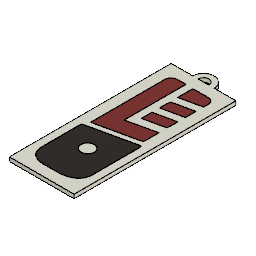
LFE (Autodesk Fusion 360 design; units mm, degrees)
Autodesk Fusion 360 part; units mm, degrees
note: some values were not read from the file. Chosen so that the rebuilt part matches the saved one: which bodies a step acts on. Set by a fixed rule: which sketch regions a step uses.
sketch "Sketch1" plane through (0, 0, 0) normal (0, 0, 1) x (1, 0, 0)
  line L0 (22.7542, -86.2542) -> (47.625, -80.8514)
  line L1 (47.625, -80.8514) -> (52.6521, -79.7322)
  line L2 (52.6521, -79.7322) -> (54.7635, -78.957)
  line L3 (54.7635, -78.957) -> (55.0333, -76.9938)
  line L4 (55.0333, -76.9938) -> (55.0333, -67.4688)
  line L5 (55.0333, -67.4688) -> (50.0063, -68.6382)
  line L6 (50.0063, -68.6382) -> (33.8667, -72.2313)
  line L7 (33.8667, -72.2313) -> (33.8667, -26.1938)
  line L8 (33.8667, -26.1938) -> (28.8396, -26.1938)
  spline S0 degree 3 poles (28.8396, -26.1938) (27.5564, -26.1964) (26.3049, -26.2176) (25.1354, -26.8393) knots 0 0 0 0 1 1 1 1
  spline S1 degree 3 poles (25.1354, -26.8393) (23.2675, -27.8315) (22.7648, -29.5196) (22.7542, -31.4854) knots 0 0 0 0 1 1 1 1
  line L9 (22.7542, -31.4854) -> (22.7542, -40.2167)
  line L10 (22.7542, -40.2167) -> (22.7542, -86.2542)
  line L11 (39.1583, -26.4583) -> (39.1583, -37.8354)
  line L12 (39.1583, -37.8354) -> (55.0333, -34.3958)
  spline S2 degree 3 poles (55.0333, -34.3958) (55.0333, -32.8057) (55.3006, -29.8979) (54.5015, -28.575) knots 0 0 0 0 1 1 1 1
  spline S3 degree 3 poles (54.5015, -28.575) (53.4485, -26.8314) (52.1626, -26.4689) (50.2708, -26.4583) knots 0 0 0 0 1 1 1 1
  line L13 (50.2708, -26.4583) -> (39.1583, -26.4583)
  line L14 (39.1583, -51.3292) -> (55.0333, -47.8896)
  line L15 (55.0333, -47.8896) -> (55.0333, -39.9521)
  line L16 (55.0333, -39.9521) -> (43.9208, -42.3016)
  line L17 (43.9208, -42.3016) -> (39.5737, -43.434)
  line L18 (39.5737, -43.434) -> (39.1583, -45.5083)
  line L19 (39.1583, -45.5083) -> (39.1583, -51.3292)
  line L20 (39.1583, -56.8854) -> (39.1583, -64.8229)
  line L21 (39.1583, -64.8229) -> (50.5354, -62.4099)
  line L22 (50.5354, -62.4099) -> (54.6179, -61.341)
  line L23 (54.6179, -61.341) -> (55.0333, -59.2667)
  line L24 (55.0333, -59.2667) -> (55.0333, -53.4458)
  line L25 (55.0333, -53.4458) -> (50.5354, -54.393)
  line L26 (50.5354, -54.393) -> (39.1583, -56.8854)
  line L27 (56.3404, -82.7114) -> (45.5083, -85.0847)
  line L28 (45.5083, -85.0847) -> (28.575, -88.8074)
  line L29 (28.575, -88.8074) -> (22.7542, -90.1118)
  spline S4 degree 3 poles (22.7542, -90.1118) (22.1377, -90.2467) (21.0344, -90.3711) (20.6428, -90.9002) knots 0 0 0 0 1 1 1 1
  spline S5 degree 3 poles (20.6428, -90.9002) (20.3121, -91.35) (20.3729, -92.3184) (20.3729, -92.8688) knots 0 0 0 0 1 1 1 1
  line L30 (20.3729, -92.8688) -> (20.3729, -112.9771)
  spline S6 degree 3 poles (20.3729, -112.9771) (20.3729, -116.2817) (20.0766, -121.322) (21.1905, -124.3542) knots 0 0 0 0 1 1 1 1
  spline S7 degree 3 poles (21.1905, -124.3542) (22.7991, -128.733) (27.0828, -130.6512) (31.4854, -130.7042) knots 0 0 0 0 1 1 1 1
  spline S8 degree 3 poles (31.4854, -130.7042) (35.8828, -130.7544) (45.1088, -131.1222) (48.9479, -129.9025) knots 0 0 0 0 1 1 1 1
  spline S9 degree 3 poles (48.9479, -129.9025) (53.9194, -128.3229) (57.4066, -125.005) (57.4146, -119.5917) knots 0 0 0 0 1 1 1 1
  line L31 (57.4146, -119.5917) -> (57.4146, -107.6854)
  line L32 (57.4146, -107.6854) -> (57.4146, -88.6354)
  line L33 (57.4146, -88.6354) -> (57.4146, -84.9313)
  spline S10 degree 3 poles (57.4146, -84.9313) (57.4146, -84.4285) (57.4754, -83.3729) (57.1447, -82.9839) knots 0 0 0 0 1 1 1 1
  spline S11 degree 3 poles (57.1447, -82.9839) (56.851, -82.6373) (56.4568, -82.7273) (56.3404, -82.7114) knots 0 0 0 0 1 1 1 1
  spline S12 degree 3 poles (37.5708, -99.3061) (38.6133, -99.2002) (39.5076, -99.2267) (40.4813, -99.6871) knots 0 0 0 0 1 1 1 1
  spline S13 degree 3 poles (40.4813, -99.6871) (45.4766, -102.0498) (43.6033, -109.3682) (38.1, -108.9819) knots 0 0 0 0 1 1 1 1
  spline S14 degree 3 poles (38.1, -108.9819) (32.6469, -108.6009) (31.7341, -100.7401) (37.5708, -99.3061) knots 0 0 0 0 1 1 1 1
  line L34 (14.7542, -18.1937) -> (63.0333, -18.1937)
  line L35 (63.0333, -18.1937) -> (63.0333, -138.7945)
  line L36 (63.0333, -138.7945) -> (14.7542, -138.7945)
  line L37 (14.7542, -138.7945) -> (14.7542, -18.1937)
  line L38 (38.0274, -130.7945) -> (16, -130.7945) construction
  circle A0 centre (38.8938, -18.1937) radius 8
  circle A1 centre (38.8938, -18.1937) radius 4
  dimension "d3" = 8
  dimension "d4" = 8
  dimension "d5" = 8
  dimension "d6" = 8
  dimension "d13" = 16
  dimension "d14" = -4
  constraint horizontal L34
  constraint vertical L35
  constraint horizontal L36
  constraint vertical L37
  constraint coincident S8 L38.start
  constraint horizontal L38
  constraint midpoint L34 A0.centre
  measures "d3" distance of L8 L34
  measures "d4" distance of L15 L35
  measures "d5" distance of L10 L37
  measures "d13" diameter of A0
extrude "Extrude1" add sketch "Sketch1" against normal blind 0.6 contours L0 L1 L2 L3 L4 L5 L6 L7 L8 S0 S1 L9 L10 | L11 L12 S2 S3 L13 | L14 L15 L16 L17 L18 L19 | L20 L21 L22 L23 L24 L25 L26 | L27 L28 L29 S4 S5 L30 S6 S7 S8 S9 L31 L32 L33 S10 S11 makes body 1 at (46.0375, -47.1734, 0) makes body 2 at (48.1542, -32.8965, 0) makes body 3 at (46.7431, -57.8961, 0) makes body 4 at (26.4583, -63.3236, 0) makes body 5 at (52.7338, -102.7556, 0)
extrude "Extrude4" add sketch "Sketch1" against normal blind 3 separate body contours L0 L1 L2 L3 L4 L5 L6 L7 L8 S0 S1 L9 L10 | L11 L12 S2 S3 L13 | L14 L15 L16 L17 L18 L19 | L20 L21 L22 L23 L24 L25 L26 | L27 L28 L29 S4 S5 L30 S6 S7 S8 S9 L31 L32 L33 S10 S11 | S12 S13 S14 | L34 A0 A1 | L34 A1 | L34 A0 A1 | L34 L35 L36 L37 A0 picked at (40.0397, -19.5366) makes body 6
combine "Combine1" operation cut target body 6 tool bodies 5 4 3 2 1 keep tools
ref_plane "WorkPlane1" through (38.776, -106.8798, -0.6) normal (0, 0, 1) x (1, 0, 0)
split "Split1" by plane through (38.776, -106.8798, -0.6) normal (0, 0, 1) bodies 6 makes body 7 at (39.6032, -136.119, 0) makes body 8 at (38.5531, -102.8878, 0)
combine "Combine2" operation add target body 6 tool bodies 7
named bodies: "LFE_keychain_tag_2", "LFE_keychain_tag_1", "LFE_keychain_tag_3", "LFE_keychain_tag_4", "LFE_keychain_tag_5", "LFE_keychain_tag_6", "LFE_keychain_tag_0"
